Autodesk Fusion 360 part; units mm, degrees
(part 2 of 3)
sketch "front-face" plane through (0, 0, 0) normal (0, 0, 1) x (1, 0, 0)
  line L0 (495.3, -266.7) -> (-495.3, -266.7)
  line L1 (-495.3, -266.7) -> (-495.3, 266.7)
  line L2 (-495.3, 266.7) -> (495.3, 266.7)
  line L3 (495.3, 266.7) -> (495.3, -266.7)
  line L4 (495.3, -266.7) -> (-495.3, 266.7) construction
  line L5 (-495.3, -266.7) -> (495.3, 266.7) construction
  line L6 (495.3, 266.7) -> (342.9, 266.7)
  line L7 (342.9, 266.7) -> (342.9, 215.9)
  line L8 (342.9, 215.9) -> (495.3, 215.9)
  line L9 (495.3, 215.9) -> (495.3, 266.7)
  line L10 (-495.3, 266.7) -> (-342.9, 266.7)
  line L11 (-342.9, 266.7) -> (-342.9, 215.9)
  line L12 (-342.9, 215.9) -> (-495.3, 215.9)
  line L13 (-495.3, 215.9) -> (-495.3, 266.7)
  line L14 (-342.9, 266.7) -> (342.9, 266.7)
  line L15 (342.9, 266.7) -> (342.9, -114.3)
  line L16 (342.9, -114.3) -> (-342.9, -114.3)
  line L17 (-342.9, -114.3) -> (-342.9, 266.7)
  line L18 (495.3, 266.7) -> (495.3, -266.7)
  line L19 (495.3, -266.7) -> (444.5, -266.7)
  line L20 (444.5, -266.7) -> (444.5, 266.7)
  line L21 (444.5, 266.7) -> (495.3, 266.7)
  line L22 (-495.3, 266.7) -> (-495.3, -266.7)
  line L23 (-495.3, -266.7) -> (-444.5, -266.7)
  line L24 (-444.5, -266.7) -> (-444.5, 266.7)
  line L25 (-444.5, 266.7) -> (-495.3, 266.7)
  line L26 (-495.3, -266.7) -> (495.3, -266.7)
  line L27 (495.3, -266.7) -> (495.3, -215.9)
  line L28 (495.3, -215.9) -> (-495.3, -215.9)
  line L29 (-495.3, -215.9) -> (-495.3, -266.7)
  line L30 (342.9, -114.3) -> (342.9, 266.7)
  line L31 (342.9, 266.7) -> (393.7, 266.7)
  line L32 (393.7, 266.7) -> (393.7, -114.3)
  line L33 (393.7, -114.3) -> (342.9, -114.3)
  line L34 (-342.9, 266.7) -> (-342.9, -114.3)
  line L35 (-342.9, -114.3) -> (-393.7, -114.3)
  line L36 (-393.7, -114.3) -> (-393.7, 266.7)
  line L37 (-393.7, 266.7) -> (-342.9, 266.7)
  line L38 (-342.9, 266.7) -> (-342.9, -114.3)
  line L39 (-342.9, -114.3) -> (-292.1, -114.3)
  line L40 (-292.1, -114.3) -> (-292.1, 266.7)
  line L41 (-292.1, 266.7) -> (-342.9, 266.7)
  line L42 (342.9, 266.7) -> (342.9, -114.3)
  line L43 (342.9, -114.3) -> (292.1, -114.3)
  line L44 (292.1, -114.3) -> (292.1, 266.7)
  line L45 (292.1, 266.7) -> (342.9, 266.7)
  line L46 (-342.9, -114.3) -> (342.9, -114.3)
  line L47 (342.9, -114.3) -> (342.9, -63.5)
  line L48 (342.9, -63.5) -> (-342.9, -63.5)
  line L49 (-342.9, -63.5) -> (-342.9, -114.3)
  line L50 (-342.9, 266.7) -> (342.9, 266.7)
  line L51 (342.9, 266.7) -> (342.9, 215.9)
  line L52 (342.9, 215.9) -> (-342.9, 215.9)
  line L53 (-342.9, 215.9) -> (-342.9, 266.7)
  line L54 (495.3, -266.7) -> (495.3, -114.3)
  line L55 (495.3, -114.3) -> (-495.3, -114.3)
  line L56 (-495.3, -114.3) -> (-495.3, -165.1)
  line L57 (-495.3, -165.1) -> (495.3, -165.1)
  line L58 (495.3, -165.1) -> (495.3, -114.3)
  line L59 (-444.5, -266.7) -> (-444.5, -215.9)
  line L60 (-444.5, -215.9) -> (-393.7, -215.9)
  line L61 (-393.7, -215.9) -> (-393.7, -266.7)
  line L62 (-393.7, -266.7) -> (-444.5, -266.7)
  line L63 (-444.5, -266.7) -> (-393.7, -215.9)
  circle A0 centre (-419.1, -241.3) radius 15.875
  circle A1 centre (-139.7, -241.3) radius 15.875
  line L64 (-165.1, -215.9) -> (-114.3, -215.9)
  line L65 (-114.3, -266.7) -> (-165.1, -266.7)
  line L66 (-165.1, -266.7) -> (-165.1, -215.9)
  line L67 (-114.3, -215.9) -> (-114.3, -266.7)
  circle A2 centre (139.7, -241.3) radius 15.875
  line L68 (114.3, -215.9) -> (165.1, -215.9)
  line L69 (165.1, -266.7) -> (114.3, -266.7)
  line L70 (114.3, -266.7) -> (114.3, -215.9)
  line L71 (165.1, -215.9) -> (165.1, -266.7)
  circle A3 centre (419.1, -241.3) radius 15.875
  line L72 (393.7, -215.9) -> (444.5, -215.9)
  line L73 (444.5, -266.7) -> (393.7, -266.7)
  line L74 (393.7, -266.7) -> (393.7, -215.9)
  line L75 (444.5, -215.9) -> (444.5, -266.7)
  line L76 (-292.1, 266.7) -> (-292.1, 215.9)
  line L77 (-292.1, 215.9) -> (-241.3, 215.9)
  line L78 (-241.3, 215.9) -> (-241.3, 266.7)
  line L79 (-241.3, 266.7) -> (-292.1, 266.7)
  line L80 (-292.1, 215.9) -> (-241.3, 266.7)
  circle A4 centre (-266.7, 241.3) radius 15.875
  line L81 (-292.1, -63.5) -> (-292.1, -114.3)
  line L82 (-292.1, -114.3) -> (-241.3, -114.3)
  line L83 (-241.3, -114.3) -> (-241.3, -63.5)
  line L84 (-241.3, -63.5) -> (-292.1, -63.5)
  line L85 (-292.1, -63.5) -> (-241.3, -114.3)
  circle A5 centre (-266.7, -88.9) radius 15.875
  circle A6 centre (-88.9, 241.3) radius 15.875
  line L86 (-63.5, 215.9) -> (-63.5, 266.7)
  line L87 (-63.5, 266.7) -> (-114.3, 266.7)
  line L88 (-114.3, 215.9) -> (-63.5, 215.9)
  line L89 (-114.3, 266.7) -> (-114.3, 215.9)
  circle A7 centre (-88.9, -88.9) radius 15.875
  line L90 (-63.5, -114.3) -> (-63.5, -63.5)
  line L91 (-63.5, -63.5) -> (-114.3, -63.5)
  line L92 (-114.3, -114.3) -> (-63.5, -114.3)
  line L93 (-114.3, -63.5) -> (-114.3, -114.3)
  circle A8 centre (88.9, 241.3) radius 15.875
  line L94 (114.3, 215.9) -> (114.3, 266.7)
  line L95 (114.3, 266.7) -> (63.5, 266.7)
  line L96 (63.5, 215.9) -> (114.3, 215.9)
  line L97 (63.5, 266.7) -> (63.5, 215.9)
  circle A9 centre (88.9, -88.9) radius 15.875
  line L98 (114.3, -114.3) -> (114.3, -63.5)
  line L99 (114.3, -63.5) -> (63.5, -63.5)
  line L100 (63.5, -114.3) -> (114.3, -114.3)
  line L101 (63.5, -63.5) -> (63.5, -114.3)
  circle A10 centre (266.7, 241.3) radius 15.875
  line L102 (292.1, 215.9) -> (292.1, 266.7)
  line L103 (292.1, 266.7) -> (241.3, 266.7)
  line L104 (241.3, 215.9) -> (292.1, 215.9)
  line L105 (241.3, 266.7) -> (241.3, 215.9)
  circle A11 centre (266.7, -88.9) radius 15.875
  line L106 (292.1, -114.3) -> (292.1, -63.5)
  line L107 (292.1, -63.5) -> (241.3, -63.5)
  line L108 (241.3, -114.3) -> (292.1, -114.3)
  line L109 (241.3, -63.5) -> (241.3, -114.3)
  line L110 (-342.9, 215.9) -> (-292.1, 215.9)
  line L111 (-292.1, 215.9) -> (-292.1, 165.1)
  line L112 (-292.1, 165.1) -> (-342.9, 165.1)
  line L113 (-342.9, 165.1) -> (-342.9, 215.9)
  line L114 (292.1, 215.9) -> (342.9, 215.9)
  line L115 (342.9, 215.9) -> (342.9, 165.1)
  line L116 (342.9, 165.1) -> (292.1, 165.1)
  line L117 (292.1, 165.1) -> (292.1, 215.9)
  line L118 (342.9, 215.9) -> (292.1, 165.1)
  line L119 (-342.9, 215.9) -> (-292.1, 165.1)
  circle A12 centre (-317.5, 190.5) radius 15.875
  circle A13 centre (317.5, 190.5) radius 15.875
  circle A14 centre (-317.5, -38.1) radius 15.875
  line L120 (-292.1, -63.5) -> (-342.9, -63.5)
  line L121 (-342.9, -63.5) -> (-342.9, -12.7)
  line L122 (-292.1, -12.7) -> (-292.1, -63.5)
  line L123 (-342.9, -12.7) -> (-292.1, -12.7)
  circle A15 centre (317.5, -38.1) radius 15.875
  line L124 (342.9, -63.5) -> (292.1, -63.5)
  line L125 (292.1, -63.5) -> (292.1, -12.7)
  line L126 (342.9, -12.7) -> (342.9, -63.5)
  line L127 (292.1, -12.7) -> (342.9, -12.7)
  line L128 (495.3, 215.9) -> (444.5, 215.9)
  line L129 (444.5, 215.9) -> (444.5, 165.1)
  line L130 (444.5, 165.1) -> (495.3, 165.1)
  line L131 (495.3, 165.1) -> (495.3, 215.9)
  line L132 (393.7, 215.9) -> (342.9, 215.9)
  line L133 (342.9, 215.9) -> (342.9, 165.1)
  line L134 (342.9, 165.1) -> (393.7, 165.1)
  line L135 (393.7, 165.1) -> (393.7, 215.9)
  line L136 (-495.3, 215.9) -> (-444.5, 215.9)
  line L137 (-444.5, 215.9) -> (-444.5, 165.1)
  line L138 (-444.5, 165.1) -> (-495.3, 165.1)
  line L139 (-495.3, 165.1) -> (-495.3, 215.9)
  line L140 (-393.7, 215.9) -> (-342.9, 215.9)
  line L141 (-342.9, 215.9) -> (-342.9, 165.1)
  line L142 (-342.9, 165.1) -> (-393.7, 165.1)
  line L143 (-393.7, 165.1) -> (-393.7, 215.9)
  line L144 (-342.9, 215.9) -> (-393.7, 165.1)
  line L145 (-495.3, 215.9) -> (-444.5, 165.1)
  line L146 (342.9, 215.9) -> (393.7, 165.1)
  line L147 (495.3, 215.9) -> (444.5, 165.1)
  circle A16 centre (469.9, 190.5) radius 15.875
  circle A17 centre (368.3, 190.5) radius 15.875
  circle A18 centre (-368.3, 190.5) radius 15.875
  circle A19 centre (-469.9, 190.5) radius 15.875
  circle A20 centre (-469.9, -88.9) radius 15.875
  line L148 (-444.5, -114.3) -> (-495.3, -114.3)
  line L149 (-342.9, -114.3) -> (-393.7, -114.3)
  circle A21 centre (-368.3, -88.9) radius 15.875
  circle A22 centre (368.3, -88.9) radius 15.875
  line L150 (342.9, -114.3) -> (393.7, -114.3)
  circle A23 centre (469.9, -88.9) radius 15.875
  line L151 (444.5, -114.3) -> (495.3, -114.3)
  line L152 (495.3, -114.3) -> (495.3, -63.5)
  line L153 (444.5, -63.5) -> (444.5, -114.3)
  line L154 (393.7, -114.3) -> (393.7, -63.5)
  line L155 (342.9, -63.5) -> (342.9, -114.3)
  line L156 (342.9, -63.5) -> (342.9, -114.3)
  line L157 (-342.9, -63.5) -> (-342.9, -114.3)
  line L158 (-342.9, -114.3) -> (-342.9, -63.5)
  line L159 (-393.7, -114.3) -> (-393.7, -63.5)
  line L160 (-444.5, -63.5) -> (-444.5, -114.3)
  line L161 (-495.3, -114.3) -> (-495.3, -63.5)
  line L162 (-495.3, -63.5) -> (-444.5, -63.5)
  line L163 (-393.7, -63.5) -> (-342.9, -63.5)
  line L164 (393.7, -63.5) -> (342.9, -63.5)
  line L165 (495.3, -63.5) -> (444.5, -63.5)
  line L166 (-495.3, -215.9) -> (-444.5, -215.9)
  line L167 (-444.5, -215.9) -> (-444.5, -165.1)
  line L168 (-444.5, -165.1) -> (-495.3, -165.1)
  line L169 (-495.3, -165.1) -> (-495.3, -215.9)
  line L170 (444.5, -215.9) -> (495.3, -215.9)
  line L171 (495.3, -215.9) -> (495.3, -165.1)
  line L172 (495.3, -165.1) -> (444.5, -165.1)
  line L173 (444.5, -165.1) -> (444.5, -215.9)
  line L174 (444.5, -215.9) -> (495.3, -165.1)
  line L175 (-444.5, -215.9) -> (-495.3, -165.1)
  circle A24 centre (-469.9, -190.5) radius 15.875
  circle A25 centre (469.9, -190.5) radius 15.875
  line L176 (495.3, -165.1) -> (342.9, -165.1)
  line L177 (342.9, -165.1) -> (292.1, -165.1)
  line L178 (292.1, -165.1) -> (292.1, -114.3)
  line L179 (292.1, -114.3) -> (342.9, -114.3)
  line L180 (342.9, -114.3) -> (342.9, -165.1)
  line L181 (342.9, -165.1) -> (292.1, -114.3)
  circle A26 centre (317.5, -139.7) radius 15.875
  circle A27 centre (105.8333, -139.7) radius 15.875
  line L182 (80.4333, -165.1) -> (80.4333, -114.3)
  line L183 (131.2333, -114.3) -> (131.2333, -165.1)
  line L184 (80.4333, -114.3) -> (131.2333, -114.3)
  line L185 (131.2333, -114.3) -> (80.4333, -114.3)
  line L186 (131.2333, -165.1) -> (80.4333, -165.1)
  circle A28 centre (-105.8333, -139.7) radius 15.875
  line L187 (-131.2333, -165.1) -> (-131.2333, -114.3)
  line L188 (-80.4333, -114.3) -> (-80.4333, -165.1)
  line L189 (-131.2333, -114.3) -> (-80.4333, -114.3)
  line L190 (-80.4333, -114.3) -> (-131.2333, -114.3)
  line L191 (-80.4333, -165.1) -> (-131.2333, -165.1)
  circle A29 centre (-317.5, -139.7) radius 15.875
  line L192 (-342.9, -165.1) -> (-342.9, -114.3)
  line L193 (-292.1, -114.3) -> (-292.1, -165.1)
  line L194 (-342.9, -114.3) -> (-292.1, -114.3)
  line L195 (-292.1, -114.3) -> (-342.9, -114.3)
  line L196 (-292.1, -165.1) -> (-342.9, -165.1)
  line L197 (495.3, 215.9) -> (444.5, 266.7)
  line L198 (342.9, 215.9) -> (393.7, 266.7)
  line L199 (-495.3, 215.9) -> (-444.5, 266.7)
  line L200 (-342.9, 215.9) -> (-393.7, 266.7)
  line L201 (-469.9, 241.3) -> (-368.3, 241.3)
  line L202 (368.3, 241.3) -> (469.9, 241.3)
  line L203 (425.45, 225.425) -> (412.75, 225.425)
  line L204 (412.75, 225.425) -> (412.75, 257.175)
  line L205 (412.75, 257.175) -> (425.45, 257.175)
  line L206 (425.45, 257.175) -> (425.45, 225.425)
  line L207 (425.45, 225.425) -> (412.75, 257.175) construction
  line L208 (412.75, 225.425) -> (425.45, 257.175) construction
  line L209 (-412.75, 225.425) -> (-425.45, 225.425)
  line L210 (-425.45, 225.425) -> (-425.45, 257.175)
  line L211 (-425.45, 257.175) -> (-412.75, 257.175)
  line L212 (-412.75, 257.175) -> (-412.75, 225.425)
  line L213 (-412.75, 225.425) -> (-425.45, 257.175) construction
  line L214 (-425.45, 225.425) -> (-412.75, 257.175) construction
  point P0 (80.4333, -114.3)
  point P1 (131.2333, -114.3)
  point P2 (131.2333, -114.3)
  point P3 (-131.2333, -114.3)
  point P4 (-80.4333, -114.3)
  point P5 (-80.4333, -114.3)
  point P6 (-342.9, -114.3)
  point P7 (-292.1, -114.3)
  point P8 (-292.1, -114.3)
  point P9 (419.1, 241.3)
  point P10 (-419.1, 241.3)
  dimension "d805" = 990.6
  dimension "d806" = 533.4
  dimension "d807" = 152.4
  dimension "d808" = 50.8
  dimension "d809" = 152.4
  dimension "d810" = 50.8
  dimension "d811" = 381
  dimension "d812" = 50.8
  dimension "d813" = 50.8
  dimension "d814" = 50.8
  dimension "d815" = 50.8
  dimension "d816" = 50.8
  dimension "d817" = 50.8
  dimension "d818" = 50.8
  dimension "d819" = 50.8
  dimension "d820" = 50.8
  dimension "d821" = 152.4
  dimension "d822" = 990.6
  dimension "d823" = 50.8
  dimension "d824" = 50.8
  dimension "d825" = 31.75
  dimension "d828" = 838.2
  dimension "d829" = 0
  dimension "d831" = 50.8
  dimension "d832" = 31.75
  dimension "d833" = 50.8
  dimension "d834" = 31.75
  dimension "d837" = 533.4
  dimension "d838" = 0
  dimension "d839" = 50.8
  dimension "d840" = 50.8
  dimension "d841" = 31.75
  dimension "d842" = 31.75
  dimension "d845" = 0
  dimension "d846" = -228.6
  dimension "d847" = 50.8
  dimension "d848" = 50.8
  dimension "d849" = 50.8
  dimension "d850" = 50.8
  dimension "d851" = 31.75
  dimension "d852" = 31.75
  dimension "d853" = 31.75
  dimension "d854" = 31.75
  dimension "d857" = 0
  dimension "d858" = -279.4
  dimension "d859" = 50.8
  dimension "d860" = 50.8
  dimension "d861" = 31.75
  dimension "d862" = 31.75
  dimension "d863" = 152.4
  dimension "d864" = 50.8
  dimension "d865" = 50.8
  dimension "d866" = 31.75
  dimension "d870" = 0
  dimension "d871" = 12.7
  dimension "d872" = 31.75
  dimension "d873" = 12.7
  dimension "d874" = 31.75
  constraint horizontal L0
  constraint perpendicular L0 L1
  constraint parallel L0 L2
  constraint parallel L1 L3
  constraint coincident L4 origin
  constraint coincident L5 origin
  constraint perpendicular L6 L7
  constraint parallel L6 L8
  constraint parallel L7 L9
  constraint perpendicular L3 L6
  constraint perpendicular L10 L11
  constraint parallel L10 L12
  constraint parallel L11 L13
  constraint perpendicular L1 L10
  constraint perpendicular L14 L15
  constraint parallel L14 L16
  constraint parallel L15 L17
  constraint perpendicular L18 L19
  constraint parallel L18 L20
  constraint parallel L19 L21
  constraint perpendicular L22 L23
  constraint parallel L22 L24
  constraint parallel L23 L25
  constraint perpendicular L26 L27
  constraint parallel L26 L28
  constraint parallel L27 L29
  constraint perpendicular L30 L31
  constraint parallel L30 L32
  constraint parallel L31 L33
  constraint perpendicular L34 L35
  constraint parallel L34 L36
  constraint parallel L35 L37
  constraint perpendicular L38 L39
  constraint parallel L38 L40
  constraint parallel L39 L41
  constraint perpendicular L42 L43
  constraint parallel L42 L44
  constraint parallel L43 L45
  constraint perpendicular L46 L47
  constraint parallel L46 L48
  constraint parallel L47 L49
  constraint perpendicular L50 L51
  constraint parallel L50 L52
  constraint parallel L51 L53
  constraint perpendicular L19 L54
  constraint horizontal L55
  constraint vertical L56
  constraint horizontal L57
  constraint vertical L58
  constraint perpendicular L59 L60
  constraint parallel L59 L61
  constraint parallel L60 L62
  constraint coincident L24 L59.end
  constraint coincident L28 L59.end
  constraint midpoint L63 A0.centre
  constraint perpendicular L76 L77
  constraint parallel L76 L78
  constraint parallel L77 L79
  constraint coincident L40 L76.end
  constraint coincident L52 L76.end
  constraint midpoint L80 A4.centre
  constraint perpendicular L81 L82
  constraint parallel L81 L83
  constraint parallel L82 L84
  constraint perpendicular L39 L81
  constraint coincident L48 L81.start
  constraint midpoint L85 A5.centre
  constraint perpendicular L110 L111
  constraint parallel L110 L112
  constraint parallel L111 L113
  constraint perpendicular L114 L115
  constraint parallel L114 L116
  constraint parallel L115 L117
  constraint midpoint L119 A12.centre
  constraint midpoint L118 A13.centre
  constraint perpendicular L128 L129
  constraint parallel L128 L130
  constraint parallel L129 L131
  constraint coincident L8 L128.end
  constraint coincident L20 L128.end
  constraint perpendicular L132 L133
  constraint parallel L132 L134
  constraint parallel L133 L135
  constraint perpendicular L7 L132
  constraint coincident L32 L132.start
  constraint perpendicular L136 L137
  constraint parallel L136 L138
  constraint parallel L137 L139
  constraint coincident L24 L136.end
  constraint coincident L12 L136.end
  constraint perpendicular L140 L141
  constraint parallel L140 L142
  constraint parallel L141 L143
  constraint perpendicular L53 L140
  constraint coincident L36 L140.start
  constraint midpoint L147 A16.centre
  constraint midpoint L146 A17.centre
  constraint midpoint L144 A18.centre
  constraint midpoint L145 A19.centre
  constraint perpendicular L166 L167
  constraint parallel L166 L168
  constraint parallel L167 L169
  constraint perpendicular L170 L171
  constraint parallel L170 L172
  constraint parallel L171 L173
  constraint midpoint L175 A24.centre
  constraint midpoint L174 A25.centre
  constraint perpendicular L171 L176
  constraint horizontal L177
  constraint vertical L178
  constraint horizontal L179
  constraint vertical L180
  constraint midpoint L181 A26.centre
  constraint midpoint L199 L201.start
  constraint midpoint L200 L201.end
  constraint midpoint L198 L202.start
  constraint midpoint L197 L202.end
  constraint horizontal L203
  constraint perpendicular L203 L204
  constraint parallel L203 L205
  constraint parallel L204 L206
  constraint coincident L207 P9
  constraint coincident L208 P9
  constraint midpoint L202 P9
  constraint horizontal L209
  constraint perpendicular L209 L210
  constraint parallel L209 L211
  constraint parallel L210 L212
  constraint coincident L213 P10
  constraint coincident L214 P10
  constraint midpoint L201 P10
  measures "d805" distance of L1.end L2.end
  measures "d806" distance of L0.end L1.end
  measures "d807" distance of L2.end L6.end
  measures "d808" distance of L6.end L7.end
  measures "d809" distance of L1.end L10.end
  measures "d810" distance of L10.end L11.end
  measures "d811" distance of L10.end P6
  measures "d812" distance of L2.end L20.end
  measures "d813" distance of L1.end L24.end
  measures "d814" distance of L0.end L28.end
  measures "d815" distance of L15.end L32.end
  measures "d816" distance of L10.end L36.end
  measures "d817" distance of L10.end L40.end
  measures "d818" distance of L6.end L44.end
  measures "d819" distance of P6 L48.end
  measures "d820" distance of L10.end L11.end
  measures "d821" distance of L0.start L54.end
  measures "d822" distance of L54.end L55.end
  measures "d823" distance of L54.end L57.end
  measures "d824" distance of L23.end L61.end
  measures "d825" diameter of A0
  measures "d831" distance of L40.end L78.end
  measures "d832" diameter of A4
  measures "d833" distance of L81.start L83.end
  measures "d834" diameter of A5
  measures "d839" distance of L11.end L112.end
  measures "d840" distance of L102.start L116.end
  measures "d841" diameter of A12
  measures "d842" diameter of A13
  measures "d847" distance of L8.end L130.end
  measures "d848" distance of L132.start L134.end
  measures "d849" distance of L12.end L138.end
  measures "d850" distance of L140.start L142.end
  measures "d851" diameter of A16
  measures "d852" diameter of A17
  measures "d853" diameter of A18
  measures "d854" diameter of A19
  measures "d859" distance of L28.end L56.end
  measures "d860" distance of L72.end L172.end
  measures "d861" diameter of A24
  measures "d862" diameter of A25
  measures "d863" distance of L57.end L176.end
  measures "d864" distance of L176.end L177.end
  measures "d865" distance of L176.end L15.end
  measures "d866" diameter of A26
  measures "d871" distance of L204.end L205.end
  measures "d872" distance of L203.end L204.end
  measures "d873" distance of L210.end L211.end
  measures "d874" distance of L209.end L210.end
extrude "Extrude16" add sketch "front-face" along normal blind 463.55 and the other way blind -457.2 separate body contours L0 L3 L18 L19 L20 L26 L27 L28 L54 L75 L170 | L0 L20 L26 L28 L72 L73 L74 L75 | L3 L18 L28 L54 L170 L171 L174 A25 | L0 L26 L28 L71 L74 | L20 L57 L172 L173 L174 A25 L176 | L3 L18 L20 L54 L55 L57 L58 L151 L172 L176 | L0 L26 L28 L68 L69 L70 L71 | L20 L33 L55 L57 L150 L176 L180 | L174 A25 | L174 A25 | L3 L18 L20 L55 L151 L152 L153 L165 | L0 L26 L28 L67 L70 | L16 L43 L46 L55 L179 L180 L181 A26 | L57 L177 L178 L181 A26 | L3 L18 L20 L130 L165 | L0 L26 L28 L64 L65 L66 L67 | L15 L30 L32 L33 L42 L47 L55 L150 L154 L155 L156 L164 | L16 L46 L55 L57 L108 L178 L183 | L181 A26 | L181 A26 | L3 L18 L130 L131 L147 A16 | L0 L26 L28 L61 L66 | L8 L20 L128 L129 L147 A16 | L15 L30 L32 L42 L126 L134 L164 | L16 L46 L55 L57 L100 L182 L183 L184 L185 L186 | L2 L3 L6 L9 L18 L21 L197 | L8 L20 L128 L197 L202 | L0 L26 L61 L62 L63 A0 | L8 L20 L32 L202 L203 L204 L206 | L147 A16 | L147 A16 | L8 L32 L132 L135 L146 A17 | L15 L30 L42 L115 L133 L134 L146 A17 | L16 L46 L55 L57 L92 L100 L182 L188 | L20 L197 L202 | L0 L1 L22 L23 L24 L26 L28 L29 L59 L166 | L24 L28 L59 L60 L63 A0 | L8 L32 L132 L198 L202 | L2 L6 L20 L32 L202 L204 L205 L206 | L146 A17 | L146 A17 | L16 L46 L55 L57 L92 L187 L188 L189 L190 L191 | L24 L57 L167 L168 L175 A24 | L1 L22 L28 L166 L169 L175 A24 | L63 A0 | L63 A0 | L2 L6 L7 L15 L30 L31 L42 L51 L198 | L32 L198 L202 | L16 L46 L55 L57 L82 L187 L193 | L1 L22 L24 L55 L56 L57 L148 L168 | L24 L35 L55 L57 L149 L192 | L175 A24 | L175 A24 | L16 L39 L46 L55 L57 L192 L193 L194 L195 L196 | L1 L22 L24 L55 L148 L160 L161 L162 | L1 L22 L24 L138 L162 | L17 L34 L35 L36 L38 L49 L55 L149 L157 L158 L159 L163 | L12 L24 L136 L137 L145 A19 | L1 L22 L138 L139 L145 A19 | L17 L34 L36 L38 L121 L142 L163 | L12 L24 L36 L201 L209 L210 L212 | L12 L24 L136 L199 L201 | L145 A19 | L145 A19 | L17 L34 L38 L113 L141 L142 L144 A18 | L12 L36 L140 L143 L144 A18 | L1 L2 L10 L13 L22 L25 L199 | L12 L36 L140 L200 L201 | L24 L199 L201 | L2 L10 L24 L36 L201 L210 L211 L212 | L144 A18 | L144 A18 | L2 L10 L11 L17 L34 L37 L38 L53 L200 | L36 L200 L201 | A1 | A2 | A3 | A20 | A21 | A22 | A23 | A27 | A28 | A29 makes body 6
extrude "Extrude17" add sketch "top-face" along normal blind 273.05 and the other way blind -266.7 separate body contours L0 L7 L23 L42 L46 L47 L48 L58 L59 L60 L66 L95 | L0 L46 L48 L60 L95 L96 | L7 L42 L48 L58 L66 L69 L71 A1 L133 L134 | L0 L46 L48 L91 L96 | L60 L67 L68 L71 A1 | L7 L42 L58 L60 L68 L74 | L0 L46 L48 L91 L92 | L71 A1 | L71 A1 | L7 L42 L52 L58 L60 L73 L74 | L7 L14 L42 L50 L51 L52 L58 L60 L61 L73 L94 L128 L184 L185 | L0 L46 L48 L87 L92 | L14 L50 L52 L60 L94 L97 | L0 L46 L48 L87 L88 | L14 L50 L52 L90 L97 L179 L180 | L0 L46 L48 L82 L88 | L14 L50 L52 L90 L93 L179 L180 | L0 L46 L81 L82 L84 A5 | L14 L50 L52 L86 L93 | L0 L11 L27 L38 L46 L48 L49 L54 L55 L56 L62 L80 | L48 L56 L80 L83 L84 A5 | L14 L50 L52 L86 L89 L174 L175 | L56 L63 L64 L70 A0 | L11 L38 L48 L54 L62 L65 L70 A0 L163 L164 | L84 A5 | L84 A5 | L14 L50 L52 L78 L89 L174 L175 | L11 L38 L54 L56 L64 L75 | L70 A0 | L70 A0 | L14 L50 L78 L79 L85 A4 | L52 L56 L76 L77 L85 A4 | L11 L38 L52 L54 L56 L72 L75 | L11 L14 L38 L50 L52 L53 L54 L56 L57 L72 L76 L144 L167 | L85 A4 | L85 A4 | A2 | A3 | A6 | A7 | A8 | A9 | A10 | A11 makes body 7
extrude "Extrude18" add sketch "front-face" along normal blind 463.55 and the other way blind -457.2 separate body contours L15 L16 L30 L42 L43 L44 L46 L47 L48 L55 L106 L124 L155 L156 L179 | L16 L44 L46 L48 L55 L106 L107 L108 L109 | L15 L30 L42 L44 L48 L124 L125 L126 L127 | L16 L46 L48 L55 L98 L109 L184 L185 | L15 L30 L42 L44 L116 L127 | L15 L30 L42 L115 L116 L118 A13 L133 | L16 L46 L48 L55 L98 L99 L100 L101 L184 L185 | L2 L7 L14 L15 L30 L42 L44 L45 L50 L51 L52 L102 L114 | L44 L52 L114 L117 L118 A13 | L16 L46 L48 L55 L90 L91 L92 L93 L189 L190 | L16 L46 L48 L55 L90 L101 | L2 L14 L44 L50 L52 L102 L103 L104 L105 | L118 A13 | L118 A13 | L16 L46 L48 L55 L83 L93 L189 L190 | L2 L14 L50 L52 L94 L105 | L16 L40 L46 L55 L81 L82 L85 A5 | L16 L17 L34 L38 L39 L40 L46 L48 L49 L55 L81 L120 L157 L158 L194 L195 | L48 L83 L84 L85 A5 | L2 L14 L50 L52 L94 L95 L96 L97 | L17 L34 L38 L40 L48 L120 L121 L122 L123 | L85 A5 | L85 A5 | L2 L14 L50 L52 L86 L97 | L17 L34 L38 L40 L112 L123 | L2 L14 L50 L52 L86 L87 L88 L89 | L40 L52 L110 L111 L119 A12 | L17 L34 L38 L112 L113 L119 A12 L141 | L2 L14 L50 L52 L78 L89 | L2 L11 L14 L17 L34 L38 L40 L41 L50 L52 L53 L76 L110 | L52 L77 L78 L80 A4 | L2 L14 L40 L50 L76 L79 L80 A4 | L119 A12 | L119 A12 | L80 A4 | L80 A4 | A6 | A7 | A8 | A9 | A10 | A11 | A14 | A15 makes body 8
sketch "LR_ribSlots" plane through (0, 0, 0) normal (1, 0, 0) x (0, 0, -1)
  line L0 (431.8, 241.3) -> (-431.8, 241.3)
  line L1 (-431.8, 241.3) -> (-431.8, -241.3)
  line L2 (-431.8, -241.3) -> (431.8, -241.3)
  line L3 (431.8, -241.3) -> (431.8, 241.3)
  line L4 (431.8, 241.3) -> (-431.8, -241.3) construction
  line L5 (-431.8, 241.3) -> (431.8, -241.3) construction
  line L6 (-415.925, -6.35) -> (-447.675, -6.35)
  line L7 (-447.675, -6.35) -> (-447.675, 6.35)
  line L8 (-447.675, 6.35) -> (-415.925, 6.35)
  line L9 (-415.925, 6.35) -> (-415.925, -6.35)
  line L10 (-415.925, -6.35) -> (-447.675, 6.35) construction
  line L11 (-447.675, -6.35) -> (-415.925, 6.35) construction
  line L12 (447.675, -6.35) -> (415.925, -6.35)
  line L13 (415.925, -6.35) -> (415.925, 6.35)
  line L14 (415.925, 6.35) -> (447.675, 6.35)
  line L15 (447.675, 6.35) -> (447.675, -6.35)
  line L16 (447.675, -6.35) -> (415.925, 6.35) construction
  line L17 (415.925, -6.35) -> (447.675, 6.35) construction
  line L18 (-431.8, 241.3) -> (-215.9, 241.3)
  line L19 (-209.55, 225.425) -> (-222.25, 225.425)
  line L20 (-222.25, 225.425) -> (-222.25, 257.175)
  line L21 (-222.25, 257.175) -> (-209.55, 257.175)
  line L22 (-209.55, 257.175) -> (-209.55, 225.425)
  line L23 (-209.55, 225.425) -> (-222.25, 257.175) construction
  line L24 (-222.25, 225.425) -> (-209.55, 257.175) construction
  line L25 (222.25, 257.175) -> (222.25, 225.425)
  line L26 (209.55, 257.175) -> (222.25, 257.175)
  line L27 (209.55, 225.425) -> (209.55, 257.175)
  line L28 (222.25, 225.425) -> (209.55, 225.425)
  line L29 (457.2, 215.9) -> (431.8, 215.9)
  line L30 (406.4, 241.3) -> (406.4, 266.7)
  line L31 (406.4, 266.7) -> (457.2, 266.7)
  line L32 (457.2, 266.7) -> (457.2, 215.9)
  line L33 (457.2, 215.9) -> (406.4, 266.7) construction
  line L34 (406.4, 215.9) -> (457.2, 266.7) construction
  line L35 (406.4, 266.7) -> (415.925, 266.7)
  line L36 (457.2, 266.7) -> (447.675, 266.7)
  line L37 (457.2, 266.7) -> (457.2, 257.175)
  line L38 (457.2, 215.9) -> (457.2, 225.425)
  line L39 (457.2, 257.175) -> (457.2, 225.425)
  line L40 (457.2, 225.425) -> (463.55, 225.425)
  line L41 (463.55, 225.425) -> (463.55, 257.175)
  line L42 (463.55, 257.175) -> (457.2, 257.175)
  line L43 (447.675, 266.7) -> (415.925, 266.7)
  line L44 (415.925, 266.7) -> (415.925, 273.05)
  line L45 (415.925, 273.05) -> (447.675, 273.05)
  line L46 (447.675, 273.05) -> (447.675, 266.7)
  line L47 (406.4, 241.3) -> (431.8, 215.9)
  line L48 (0, 241.3) -> (0, -241.3)
  line L49 (-406.4, 241.3) -> (-431.8, 215.9)
  line L50 (-457.2, 215.9) -> (-431.8, 215.9)
  line L51 (-457.2, 215.9) -> (-457.2, 225.425)
  line L52 (-457.2, 225.425) -> (-463.55, 225.425)
  line L53 (-463.55, 225.425) -> (-463.55, 257.175)
  line L54 (-463.55, 257.175) -> (-457.2, 257.175)
  line L55 (-457.2, 266.7) -> (-457.2, 257.175)
  line L56 (-457.2, 266.7) -> (-447.675, 266.7)
  line L57 (-447.675, 273.05) -> (-447.675, 266.7)
  line L58 (-415.925, 273.05) -> (-447.675, 273.05)
  line L59 (-415.925, 266.7) -> (-415.925, 273.05)
  line L60 (-406.4, 266.7) -> (-415.925, 266.7)
  line L61 (-406.4, 241.3) -> (-406.4, 266.7)
  point P0 (-431.8, 0)
  point P1 (431.8, 0)
  point P2 (-215.9, 241.3)
  point P3 (215.9, 241.3)
  point P4 (431.8, 241.3)
  dimension "d688" = 863.6
  dimension "d689" = 482.6
  dimension "d690" = 31.75
  dimension "d691" = 12.7
  dimension "d692" = 31.75
  dimension "d693" = 12.7
  dimension "d694" = 215.9
  dimension "d695" = 12.7
  dimension "d696" = 31.75
  dimension "d699" = 431.8
  dimension "d700" = 0
  dimension "d779" = 50.8
  dimension "d780" = 50.8
  dimension "d781" = 9.525
  dimension "d782" = 9.525
  dimension "d783" = 9.525
  dimension "d784" = 9.525
  dimension "d785" = 6.35
  dimension "d786" = 6.35
  dimension "d787" = 25.4
  dimension "d788" = 25.4
  constraint horizontal L0
  constraint perpendicular L0 L1
  constraint parallel L0 L2
  constraint parallel L1 L3
  constraint coincident L4 origin
  constraint coincident L5 origin
  constraint horizontal L6
  constraint perpendicular L6 L7
  constraint parallel L6 L8
  constraint parallel L7 L9
  constraint coincident L10 P0
  constraint coincident L11 P0
  constraint midpoint L1 P0
  constraint horizontal L12
  constraint perpendicular L12 L13
  constraint parallel L12 L14
  constraint parallel L13 L15
  constraint coincident L16 P1
  constraint coincident L17 P1
  constraint midpoint L3 P1
  constraint perpendicular L3 L18
  constraint horizontal L19
  constraint perpendicular L19 L20
  constraint parallel L19 L21
  constraint parallel L20 L22
  constraint coincident L23 P2
  constraint coincident L24 P2
  constraint coincident P2 L18.end
  constraint horizontal L29
  constraint perpendicular L29 L30
  constraint parallel L29 L31
  constraint parallel L30 L32
  constraint coincident L33 P4
  constraint coincident L34 P4
  constraint coincident P4 L0.start
  constraint perpendicular L32 L36
  constraint perpendicular L31 L37
  constraint perpendicular L29 L38
  constraint perpendicular L39 L40
  constraint parallel L39 L41
  constraint parallel L40 L42
  constraint perpendicular L43 L44
  constraint parallel L43 L45
  constraint parallel L44 L46
  constraint parallel L31 L43
  constraint coincident L34.start L30
  constraint coincident L34.start L29
  constraint midpoint L0 L48.start
  constraint midpoint L2 L48.end
  constraint symmetric L29.start L48 L50.start
  constraint symmetric L30.end L48 L60.start
  constraint symmetric L31.end L48 L55.start
  constraint symmetric L35.end L48 L59.start
  constraint symmetric L36.end L48 L56.end
  constraint symmetric L37.end L48 L54.end
  constraint symmetric L38.end L48 L51.end
  constraint symmetric L40.end L48 L52.end
  constraint symmetric L41.end L48 L53.end
  constraint symmetric L44.end L48 L58.start
  constraint symmetric L45.end L48 L57.start
  constraint symmetric L30.start L48 L49.start
  constraint symmetric L29.end L48 L49.end
  measures "d688" distance of L1.end L2.end
  measures "d689" distance of L0.end L1.end
  measures "d690" distance of L7.end L8.end
  measures "d691" distance of L6.end L7.end
  measures "d692" distance of L13.end L14.end
  measures "d693" distance of L12.end L13.end
  measures "d694" distance of L0.end L18.end
  measures "d695" distance of L20.end L21.end
  measures "d696" distance of L19.end L20.end
  measures "d779" distance of L30.end L31.end
  measures "d780" distance of L34.start L30.end
  measures "d781" distance of L30.end L35.end
  measures "d782" distance of L31.end L36.end
  measures "d783" distance of L31.end L37.end
  measures "d784" distance of L29.start L38.end
  measures "d785" distance of L37.end L41.end
  measures "d786" distance of L36.end L45.end
  measures "d787" distance of L34.start L30.start
  measures "d788" distance of L34.start L29.end
extrude "Extrude21" cut sketch "LR_ribSlots" along normal mid plane 1003.3 contours L0 L25 L27 L28 | L0 L25 L26 L27 | L3 L12 L14 L15 | L3 L12 L13 L14 | L0 L18 L19 L20 L22 | L0 L18 L20 L21 L22 | L1 L6 L7 L8 | L1 L6 L8 L9 bodies 3 4
sketch "top_ribSlots" plane through (0, 0, 0) normal (0, 1, 0) x (1, 0, 0)
  line L0 (469.9, 431.8) -> (-469.9, 431.8)
  line L1 (-469.9, 431.8) -> (-469.9, -431.8)
  line L2 (-469.9, -431.8) -> (469.9, -431.8)
  line L3 (469.9, -431.8) -> (469.9, 431.8)
  line L4 (469.9, 431.8) -> (-469.9, -431.8) construction
  line L5 (-469.9, 431.8) -> (469.9, -431.8) construction
  line L6 (469.9, -431.8) -> (469.9, -215.9)
  line L7 (-469.9, -431.8) -> (-469.9, -215.9)
  line L8 (-469.9, 431.8) -> (-234.95, 431.8)
  line L9 (-241.3, 447.675) -> (-228.6, 447.675)
  line L10 (-228.6, 447.675) -> (-228.6, 415.925)
  line L11 (-228.6, 415.925) -> (-241.3, 415.925)
  line L12 (-241.3, 415.925) -> (-241.3, 447.675)
  line L13 (-241.3, 447.675) -> (-228.6, 415.925) construction
  line L14 (-228.6, 447.675) -> (-241.3, 415.925) construction
  line L15 (-485.775, -209.55) -> (-454.025, -209.55)
  line L16 (-454.025, -209.55) -> (-454.025, -222.25)
  line L17 (-454.025, -222.25) -> (-485.775, -222.25)
  line L18 (-485.775, -222.25) -> (-485.775, -209.55)
  line L19 (-485.775, -209.55) -> (-454.025, -222.25) construction
  line L20 (-454.025, -209.55) -> (-485.775, -222.25) construction
  line L21 (454.025, -209.55) -> (485.775, -209.55)
  line L22 (485.775, -209.55) -> (485.775, -222.25)
  line L23 (485.775, -222.25) -> (454.025, -222.25)
  line L24 (454.025, -222.25) -> (454.025, -209.55)
  line L25 (454.025, -209.55) -> (485.775, -222.25) construction
  line L26 (485.775, -209.55) -> (454.025, -222.25) construction
  line L27 (454.025, 222.25) -> (485.775, 222.25)
  line L28 (454.025, 209.55) -> (454.025, 222.25)
  line L29 (485.775, 209.55) -> (454.025, 209.55)
  line L30 (485.775, 222.25) -> (485.775, 209.55)
  line L31 (-485.775, 222.25) -> (-454.025, 222.25)
  line L32 (-485.775, 209.55) -> (-485.775, 222.25)
  line L33 (-454.025, 209.55) -> (-485.775, 209.55)
  line L34 (-454.025, 222.25) -> (-454.025, 209.55)
  line L35 (241.3, 415.925) -> (228.6, 415.925)
  line L36 (228.6, 415.925) -> (228.6, 447.675)
  line L37 (228.6, 447.675) -> (241.3, 447.675)
  line L38 (241.3, 447.675) -> (241.3, 415.925)
  line L39 (495.3, -406.4) -> (469.9, -406.4)
  line L40 (444.5, -431.8) -> (444.5, -457.2)
  line L41 (444.5, -457.2) -> (495.3, -457.2)
  line L42 (495.3, -457.2) -> (495.3, -406.4)
  line L43 (495.3, -406.4) -> (444.5, -457.2) construction
  line L44 (444.5, -406.4) -> (495.3, -457.2) construction
  line L45 (444.5, -457.2) -> (454.025, -457.2)
  line L46 (495.3, -406.4) -> (495.3, -415.925)
  line L47 (495.3, -457.2) -> (495.3, -447.675)
  line L48 (495.3, -457.2) -> (485.775, -457.2)
  line L49 (495.3, -447.675) -> (495.3, -415.925)
  line L50 (495.3, -415.925) -> (501.65, -415.925)
  line L51 (501.65, -415.925) -> (501.65, -447.675)
  line L52 (501.65, -447.675) -> (495.3, -447.675)
  line L53 (485.775, -457.2) -> (454.025, -457.2)
  line L54 (454.025, -457.2) -> (454.025, -463.55)
  line L55 (454.025, -463.55) -> (485.775, -463.55)
  line L56 (485.775, -463.55) -> (485.775, -457.2)
  line L57 (469.9, 0) -> (-469.9, 0)
  line L58 (0, 431.8) -> (0, -431.8)
  line L59 (469.9, -406.4) -> (444.5, -431.8)
  line L60 (-469.9, -406.4) -> (-444.5, -431.8)
  line L61 (-444.5, -431.8) -> (-444.5, -457.2)
  line L62 (-444.5, -457.2) -> (-454.025, -457.2)
  line L63 (-454.025, -457.2) -> (-454.025, -463.55)
  line L64 (-454.025, -463.55) -> (-485.775, -463.55)
  line L65 (-485.775, -463.55) -> (-485.775, -457.2)
  line L66 (-495.3, -406.4) -> (-469.9, -406.4)
  line L67 (-495.3, -406.4) -> (-495.3, -415.925)
  line L68 (-495.3, -415.925) -> (-501.65, -415.925)
  line L69 (-501.65, -415.925) -> (-501.65, -447.675)
  line L70 (-501.65, -447.675) -> (-495.3, -447.675)
  line L71 (-495.3, -457.2) -> (-495.3, -447.675)
  line L72 (-495.3, -457.2) -> (-485.775, -457.2)
  line L73 (469.9, 406.4) -> (444.5, 431.8)
  line L74 (495.3, 406.4) -> (469.9, 406.4)
  line L75 (495.3, 406.4) -> (495.3, 415.925)
  line L76 (495.3, 415.925) -> (501.65, 415.925)
  line L77 (501.65, 415.925) -> (501.65, 447.675)
  line L78 (444.5, 431.8) -> (444.5, 457.2)
  line L79 (444.5, 457.2) -> (454.025, 457.2)
  line L80 (454.025, 457.2) -> (454.025, 463.55)
  line L81 (454.025, 463.55) -> (485.775, 463.55)
  line L82 (485.775, 463.55) -> (485.775, 457.2)
  line L83 (495.3, 457.2) -> (485.775, 457.2)
  line L84 (495.3, 457.2) -> (495.3, 447.675)
  line L85 (501.65, 447.675) -> (495.3, 447.675)
  line L86 (-469.9, 406.4) -> (-444.5, 431.8)
  line L87 (-444.5, 431.8) -> (-444.5, 457.2)
  line L88 (-495.3, 406.4) -> (-469.9, 406.4)
  line L89 (-495.3, 406.4) -> (-495.3, 415.925)
  line L90 (-495.3, 415.925) -> (-501.65, 415.925)
  line L91 (-501.65, 415.925) -> (-501.65, 447.675)
  line L92 (-501.65, 447.675) -> (-495.3, 447.675)
  line L93 (-495.3, 457.2) -> (-495.3, 447.675)
  line L94 (-495.3, 457.2) -> (-485.775, 457.2)
  line L95 (-485.775, 463.55) -> (-485.775, 457.2)
  line L96 (-444.5, 457.2) -> (-454.025, 457.2)
  line L97 (-454.025, 457.2) -> (-454.025, 463.55)
  line L98 (-454.025, 463.55) -> (-485.775, 463.55)
  point P0 (-234.95, 431.8)
  point P1 (-469.9, -215.9)
  point P2 (469.9, -215.9)
  point P3 (469.9, 215.9)
  point P4 (234.95, 431.8)
  point P5 (469.9, -431.8)
  dimension "d703" = 939.8
  dimension "d704" = 863.6
  dimension "d705" = 215.9
  dimension "d706" = 215.9
  dimension "d707" = 234.95
  dimension "d708" = 12.7
  dimension "d709" = 31.75
  dimension "d710" = 31.75
  dimension "d711" = 12.7
  dimension "d712" = 31.75
  dimension "d713" = 12.7
  dimension "d716" = 0
  dimension "d717" = 431.8
  dimension "d720" = 469.9
  dimension "d721" = 0
  dimension "d749" = 50.8
  dimension "d750" = 50.8
  dimension "d751" = 9.525
  dimension "d752" = 9.525
  dimension "d753" = 9.525
  dimension "d754" = 9.525
  dimension "d755" = 6.35
  dimension "d756" = 6.35
  dimension "d757" = 25.4
  dimension "d758" = 25.4
  constraint horizontal L0
  constraint perpendicular L0 L1
  constraint parallel L0 L2
  constraint parallel L1 L3
  constraint coincident L4 origin
  constraint coincident L5 origin
  constraint perpendicular L2 L6
  constraint perpendicular L2 L7
  constraint perpendicular L1 L8
  constraint horizontal L9
  constraint perpendicular L9 L10
  constraint parallel L9 L11
  constraint parallel L10 L12
  constraint coincident L13 P0
  constraint coincident L14 P0
  constraint coincident P0 L8.end
  constraint horizontal L15
  constraint perpendicular L15 L16
  constraint parallel L15 L17
  constraint parallel L16 L18
  constraint coincident L19 P1
  constraint coincident L20 P1
  constraint coincident P1 L7.end
  constraint horizontal L21
  constraint perpendicular L21 L22
  constraint parallel L21 L23
  constraint parallel L22 L24
  constraint coincident L25 P2
  constraint coincident L26 P2
  constraint coincident P2 L6.end
  constraint horizontal L39
  constraint perpendicular L39 L40
  constraint parallel L39 L41
  constraint parallel L40 L42
  constraint coincident L43 P5
  constraint coincident L44 P5
  constraint coincident P5 L2.end
  constraint perpendicular L40 L45
  constraint perpendicular L39 L46
  constraint perpendicular L41 L47
  constraint perpendicular L42 L48
  constraint perpendicular L49 L50
  constraint parallel L49 L51
  constraint parallel L50 L52
  constraint perpendicular L53 L54
  constraint parallel L53 L55
  constraint parallel L54 L56
  constraint midpoint L3 L57.start
  constraint midpoint L1 L57.end
  constraint midpoint L0 L58.start
  constraint midpoint L2 L58.end
  constraint coincident L44.start L39
  constraint coincident L44.start L40
  constraint symmetric L39.start L58 L66.start
  constraint symmetric L40.end L58 L61.end
  constraint symmetric L41.end L58 L71.start
  constraint symmetric L45.end L58 L62.end
  constraint symmetric L46.end L58 L67.end
  constraint symmetric L47.end L58 L70.end
  constraint symmetric L48.end L58 L65.end
  constraint symmetric L50.end L58 L68.end
  constraint symmetric L51.end L58 L69.end
  constraint symmetric L54.end L58 L63.end
  constraint symmetric L55.end L58 L64.end
  constraint symmetric L58 L39.end L60.start
  constraint symmetric L58 L40.start L60.end
  constraint symmetric L39.start L57 L74.start
  constraint symmetric L40.end L57 L78.end
  constraint symmetric L41.end L57 L83.start
  constraint symmetric L45.end L57 L79.end
  constraint symmetric L46.end L57 L75.end
  constraint symmetric L47.end L57 L84.end
  constraint symmetric L48.end L57 L82.end
  constraint symmetric L50.end L57 L76.end
  constraint symmetric L51.end L57 L77.end
  constraint symmetric L54.end L57 L80.end
  constraint symmetric L55.end L57 L81.end
  constraint symmetric L57 L39.end L73.start
  constraint symmetric L57 L40.start L73.end
  constraint symmetric L57 L60.start L86.start
  constraint symmetric L57 L60.end L86.end
  constraint symmetric L57 L61.end L87.end
  constraint symmetric L57 L62.end L96.end
  constraint symmetric L57 L63.end L97.end
  constraint symmetric L57 L64.end L95.start
  constraint symmetric L57 L65.end L94.end
  constraint symmetric L57 L66.start L88.start
  constraint symmetric L57 L67.end L89.end
  constraint symmetric L57 L68.end L90.end
  constraint symmetric L57 L69.end L91.end
  constraint symmetric L57 L70.end L92.end
  constraint symmetric L57 L71.start L93.start
  measures "d703" distance of L1.end P5
  measures "d704" distance of L0.end L1.end
  measures "d705" distance of P5 P2
  measures "d706" distance of L1.end P1
  measures "d707" distance of L0.end P0
  measures "d708" distance of L10.end L11.end
  measures "d709" distance of L9.end L10.end
  measures "d710" distance of L16.end L17.end
  measures "d711" distance of L15.end L16.end
  measures "d712" distance of L22.end L23.end
  measures "d713" distance of L21.end L22.end
  measures "d749" distance of L40.end L41.end
  measures "d750" distance of L44.start L40.end
  measures "d751" distance of L40.end L45.end
  measures "d752" distance of L39.start L46.end
  measures "d753" distance of L41.end L47.end
  measures "d754" distance of L41.end L48.end
  measures "d755" distance of L47.end L51.end
  measures "d756" distance of L48.end L55.end
  measures "d757" distance of L44.start L39.end
  measures "d758" distance of L44.start L40.start
extrude "Extrude22" cut sketch "top_ribSlots" along normal blind 273.05 contours L0 L35 L36 L38 | L0 L36 L37 L38 | L3 L27 L29 L30 | L3 L27 L28 L29 | L0 L8 L10 L11 L12 | L0 L8 L9 L10 L12 | L3 L6 L21 L22 L23 | L3 L6 L21 L23 L24 | L1 L31 L32 L33 | L1 L31 L33 L34 | L1 L7 L15 L16 L17 | L1 L7 L15 L17 L18 bodies 5
sketch "front/back_ribSlots" plane through (0, 0, 0) normal (0, 0, 1) x (1, 0, 0)
  line L0 (469.9, 241.3) -> (-469.9, 241.3)
  line L1 (-469.9, 241.3) -> (-469.9, -241.3)
  line L2 (-469.9, -241.3) -> (469.9, -241.3)
  line L3 (469.9, -241.3) -> (469.9, 241.3)
  line L4 (469.9, 241.3) -> (-469.9, -241.3) construction
  line L5 (-469.9, 241.3) -> (469.9, -241.3) construction
  line L6 (469.9, 241.3) -> (234.95, 241.3)
  line L7 (228.6, 225.425) -> (241.3, 225.425)
  line L8 (241.3, 225.425) -> (241.3, 257.175)
  line L9 (241.3, 257.175) -> (228.6, 257.175)
  line L10 (228.6, 257.175) -> (228.6, 225.425)
  line L11 (228.6, 225.425) -> (241.3, 257.175) construction
  line L12 (241.3, 225.425) -> (228.6, 257.175) construction
  line L13 (454.025, 6.35) -> (485.775, 6.35)
  line L14 (485.775, 6.35) -> (485.775, -6.35)
  line L15 (485.775, -6.35) -> (454.025, -6.35)
  line L16 (454.025, -6.35) -> (454.025, 6.35)
  line L17 (454.025, 6.35) -> (485.775, -6.35) construction
  line L18 (485.775, 6.35) -> (454.025, -6.35) construction
  line L19 (-485.775, -6.35) -> (-454.025, -6.35)
  line L20 (-454.025, -6.35) -> (-454.025, 6.35)
  line L21 (-454.025, 6.35) -> (-485.775, 6.35)
  line L22 (-485.775, 6.35) -> (-485.775, -6.35)
  line L23 (-485.775, -6.35) -> (-454.025, 6.35) construction
  line L24 (-454.025, -6.35) -> (-485.775, 6.35) construction
  line L25 (-241.3, 257.175) -> (-241.3, 225.425)
  line L26 (-228.6, 257.175) -> (-241.3, 257.175)
  line L27 (-228.6, 225.425) -> (-228.6, 257.175)
  line L28 (-241.3, 225.425) -> (-228.6, 225.425)
  line L29 (-495.3, 215.9) -> (-469.9, 215.9)
  line L30 (-444.5, 241.3) -> (-444.5, 266.7)
  line L31 (-444.5, 266.7) -> (-495.3, 266.7)
  line L32 (-495.3, 266.7) -> (-495.3, 215.9)
  line L33 (-495.3, 215.9) -> (-444.5, 266.7) construction
  line L34 (-444.5, 215.9) -> (-495.3, 266.7) construction
  line L35 (-495.3, 266.7) -> (-495.3, 257.175)
  line L36 (-495.3, 266.7) -> (-485.775, 266.7)
  line L37 (-444.5, 266.7) -> (-454.025, 266.7)
  line L38 (-495.3, 215.9) -> (-495.3, 225.425)
  line L39 (-454.025, 266.7) -> (-485.775, 266.7)
  line L40 (-485.775, 266.7) -> (-485.775, 273.05)
  line L41 (-485.775, 273.05) -> (-454.025, 273.05)
  line L42 (-454.025, 273.05) -> (-454.025, 266.7)
  line L43 (-495.3, 257.175) -> (-495.3, 225.425)
  line L44 (-495.3, 225.425) -> (-501.65, 225.425)
  line L45 (-501.65, 225.425) -> (-501.65, 257.175)
  line L46 (-501.65, 257.175) -> (-495.3, 257.175)
  line L47 (-444.5, 241.3) -> (-469.9, 215.9)
  line L48 (0, 241.3) -> (0, -241.3)
  line L49 (444.5, 241.3) -> (469.9, 215.9)
  line L50 (444.5, 241.3) -> (444.5, 266.7)
  line L51 (495.3, 215.9) -> (469.9, 215.9)
  line L52 (495.3, 215.9) -> (495.3, 225.425)
  line L53 (495.3, 225.425) -> (501.65, 225.425)
  line L54 (501.65, 225.425) -> (501.65, 257.175)
  line L55 (501.65, 257.175) -> (495.3, 257.175)
  line L56 (495.3, 266.7) -> (495.3, 257.175)
  line L57 (495.3, 266.7) -> (485.775, 266.7)
  line L58 (485.775, 266.7) -> (485.775, 273.05)
  line L59 (485.775, 273.05) -> (454.025, 273.05)
  line L60 (454.025, 273.05) -> (454.025, 266.7)
  line L61 (444.5, 266.7) -> (454.025, 266.7)
  point P0 (234.95, 241.3)
  point P1 (469.9, 0)
  point P2 (-469.9, 0)
  point P3 (-234.95, 241.3)
  point P4 (-469.9, 241.3)
  dimension "d724" = 939.8
  dimension "d725" = 482.6
  dimension "d726" = 234.95
  dimension "d727" = 12.7
  dimension "d728" = 31.75
  dimension "d729" = 31.75
  dimension "d730" = 12.7
  dimension "d731" = 31.75
  dimension "d732" = 12.7
  dimension "d735" = -469.9
  dimension "d736" = 0
  dimension "d761" = 50.8
  dimension "d762" = 50.8
  dimension "d763" = 9.525
  dimension "d764" = 9.525
  dimension "d765" = 9.525
  dimension "d766" = 9.525
  dimension "d767" = 6.35
  dimension "d768" = 6.35
  dimension "d769" = 25.4
  dimension "d770" = 25.4
  constraint horizontal L0
  constraint perpendicular L0 L1
  constraint parallel L0 L2
  constraint parallel L1 L3
  constraint coincident L4 origin
  constraint coincident L5 origin
  constraint perpendicular L3 L6
  constraint horizontal L7
  constraint perpendicular L7 L8
  constraint parallel L7 L9
  constraint parallel L8 L10
  constraint coincident L11 P0
  constraint coincident L12 P0
  constraint coincident P0 L6.end
  constraint horizontal L13
  constraint perpendicular L13 L14
  constraint parallel L13 L15
  constraint parallel L14 L16
  constraint coincident L17 P1
  constraint coincident L18 P1
  constraint midpoint L3 P1
  constraint horizontal L19
  constraint perpendicular L19 L20
  constraint parallel L19 L21
  constraint parallel L20 L22
  constraint coincident L23 P2
  constraint coincident L24 P2
  constraint midpoint L1 P2
  constraint horizontal L29
  constraint perpendicular L29 L30
  constraint parallel L29 L31
  constraint parallel L30 L32
  constraint coincident L33 P4
  constraint coincident L34 P4
  constraint coincident P4 L0.end
  constraint perpendicular L31 L35
  constraint perpendicular L32 L36
  constraint perpendicular L30 L37
  constraint perpendicular L29 L38
  constraint perpendicular L39 L40
  constraint parallel L39 L41
  constraint parallel L40 L42
  constraint perpendicular L43 L44
  constraint parallel L43 L45
  constraint parallel L44 L46
  constraint coincident L34.start L30
  constraint coincident L34.start L29
  constraint midpoint L0 L48.start
  constraint midpoint L2 L48.end
  constraint symmetric L29.start L48 L51.start
  constraint symmetric L30.end L48 L50.end
  constraint symmetric L31.end L48 L56.start
  constraint symmetric L35.end L48 L55.end
  constraint symmetric L36.end L48 L57.end
  constraint symmetric L37.end L48 L60.end
  constraint symmetric L38.end L48 L52.end
  constraint symmetric L40.end L48 L58.end
  constraint symmetric L41.end L48 L59.end
  constraint symmetric L44.end L48 L53.end
  constraint symmetric L45.end L48 L54.end
  constraint symmetric L30.start L48 L49.start
  constraint symmetric L29.end L48 L49.end
  measures "d724" distance of L1.end L2.end
  measures "d725" distance of P4 L1.end
  measures "d726" distance of L0.start P0
  measures "d727" distance of L8.end L9.end
  measures "d728" distance of L7.end L8.end
  measures "d729" distance of L14.end L15.end
  measures "d730" distance of L13.end L14.end
  measures "d731" distance of L20.end L21.end
  measures "d732" distance of L19.end L20.end
  measures "d761" distance of L30.end L31.end
  measures "d762" distance of L34.start L30.end
  measures "d763" distance of L31.end L35.end
  measures "d764" distance of L31.end L36.end
  measures "d765" distance of L30.end L37.end
  measures "d766" distance of L29.start L38.end
  measures "d767" distance of L37.end L41.end
  measures "d768" distance of L35.end L45.end
  measures "d769" distance of L34.start L30.start
  measures "d770" distance of L34.start L29.end
extrude "Extrude23" cut sketch "front/back_ribSlots" along normal mid plane 927.1 contours L3 L13 L14 L15 | L3 L13 L15 L16 | L1 L19 L21 L22 | L1 L19 L20 L21 bodies 2 6